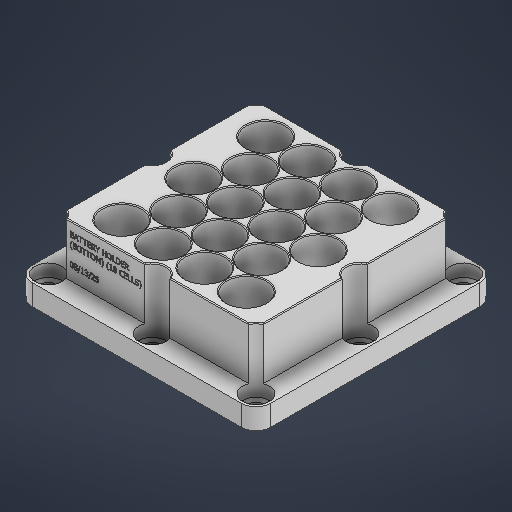
# Autodesk Inventor part: Battery Holder
Saved by Autodesk Inventor 2025 (Build 290162000, 162)
## iProperties
Created: 2025-08-08
Part Number: Battery Holder
Material: Generic
Document SubType Name: Modeling
Designer: mayhe
Density: 1 g/cm^3
Appearance: Default
Author: mayhe
Autodesk Inventor part; units mm, degrees
ref_plane "YZ Plane" through (0, 0, 0) normal (1, 0, 0) x (0, 1, 0)
ref_plane "XZ Plane" through (0, 0, 0) normal (0, 1, 0) x (-1, 0, 0)
ref_plane "XY Plane" through (0, 0, 0) normal (0, 0, 1) x (1, 0, 0)
sketch "Sketch1" plane through (0, 0, 0) normal (0, 1, 0) x (-1, 0, 0)
  line L0 (57.5, 57.5) -> (-57.5, 57.5)
  line L1 (-57.5, 57.5) -> (-57.5, -57.5)
  line L2 (-57.5, -57.5) -> (57.5, -57.5)
  line L3 (57.5, -57.5) -> (57.5, 57.5)
  line L4 (57.5, 57.5) -> (-57.5, -57.5) construction
  line L5 (-57.5, 57.5) -> (57.5, -57.5) construction
  point P0 (0, 0)
  dimension "d0" = 115
  dimension "d1" = 115
  constraints: 12 end point, 2 midpoint, 2 parallel, 1 horizontal, 1 perpendicular
  measures "d0" distance of L2.end L1.end
  measures "d1" distance of L1.end L0.end
extrude "Extrusion1" add sketch "Sketch1" along normal blind 10
sketch "Sketch4" plane through (0, 10, 0) normal (0, 1, 0) x (1, 0, 0)
  line L0 (-47.5, -47.5) -> (47.5, -47.5)
  line L1 (47.5, -47.5) -> (47.5, 47.5)
  line L2 (47.5, 47.5) -> (-47.5, 47.5)
  line L3 (-47.5, 47.5) -> (-47.5, -47.5)
  line L4 (-57.5, 57.5) -> (-57.5, -57.5) projected
  line L5 (-57.5, 0) -> (-47.5, 0)
  line L6 (-30, 34.641) -> (30, 34.641)
  line L7 (30, 34.641) -> (30, -34.641)
  line L8 (30, -34.641) -> (-30, -34.641)
  line L9 (-30, -34.641) -> (-30, 34.641)
  line L10 (-30, 34.641) -> (30, -34.641) construction
  line L11 (30, 34.641) -> (-30, -34.641) construction
  circle A0 centre (-30, 34.641) radius 9.5
  circle A1 centre (-10, 34.641) radius 9.5
  circle A2 centre (10, 34.641) radius 9.5
  circle A3 centre (30, 34.641) radius 9.5
  circle A4 centre (-30, 0) radius 9.5
  circle A5 centre (-10, 0) radius 9.5
  circle A6 centre (10, 0) radius 9.5
  circle A7 centre (30, 0) radius 9.5
  circle A8 centre (-30, -34.641) radius 9.5
  circle A9 centre (-10, -34.641) radius 9.5
  circle A10 centre (10, -34.641) radius 9.5
  circle A11 centre (30, -34.641) radius 9.5
  circle A12 centre (-20, 17.3205) radius 9.5
  circle A13 centre (0, 17.3205) radius 9.5
  circle A14 centre (20, 17.3205) radius 9.5
  circle A15 centre (-20, -17.3205) radius 9.5
  circle A16 centre (0, -17.3205) radius 9.5
  circle A17 centre (20, -17.3205) radius 9.5
  point P0 (47.3285, -94.6135)
  point P1 (-53.5957, 219.1108)
  point P2 (0, 0)
  dimension "d1" = 115
  dimension "d138" = 3
  dimension "d48" = 95
  dimension "d49" = 95
  dimension "d132" = 60
  dimension "d133" = 69.282
  dimension "d134" = 19
  dimension "d137" = 20
  dimension "d140" = 34.641
  dimension "d143" = 19
  dimension "d146" = 10
  dimension "d147" = 17.3205
  dimension "d150" = 20
  dimension "d153" = 34.641
  constraints: 22 end point, 18 centre point, 4 horizontal, 4 midpoint, 4 parallel, 2 perpendicular, 2 vertical, 1 coincident, 32 other
  measures "d48" distance of L2.end L1.end
  measures "d49" distance of L1.end L0.end
  measures "d132" distance of L7.end L8.end
  measures "d133" distance of L6.end L7.end
  measures "d134" diameter of A0
  measures "d137" distance of A0.centre A1.centre
  measures "d140" distance of A0.centre A4.centre
  measures "d143" diameter of A12
  measures "d146" horizontal distance of A1.centre A12.centre
  measures "d147" vertical distance of A12.centre A1.centre
  measures "d150" distance of A12.centre A13.centre
  measures "d153" distance of A12.centre A15.centre
extrude "Extrusion2" add sketch "Sketch4" along normal blind 25 contours L3 L2 L1 L0 | L6 A1 A2 A3 L7 A7 A11 L8 A10 A9 A8 L9 A4 A0
sketch "Sketch5" plane through (0, 35, 0) normal (0, 1, 0) x (1, 0, 0)
  line L0 (50, 50) -> (-50, 50)
  line L1 (-50, 50) -> (-50, -50)
  line L2 (-50, -50) -> (50, -50)
  line L3 (50, -50) -> (50, 50)
  line L4 (50, 50) -> (-50, -50) construction
  line L5 (-50, 50) -> (50, -50) construction
  circle A0 centre (-50, -50) radius 3.5
  circle A1 centre (0, -50) radius 3.5
  circle A2 centre (-50, 0) radius 3.5
  circle A3 centre (0, 0) radius 3.5
  circle A4 centre (50, -50) radius 3.5
  circle A5 centre (50, 0) radius 3.5
  circle A6 centre (-50, 50) radius 3.5
  circle A7 centre (0, 50) radius 3.5
  circle A8 centre (50, 50) radius 3.5
  point P0 (0, 0)
  dimension "d156" = 100
  dimension "d157" = 100
  dimension "d158" = 7
  dimension "d161" = 50
  dimension "d164" = 50
  constraints: 12 end point, 9 centre point, 2 horizontal, 2 midpoint, 2 parallel, 1 coincident, 1 perpendicular, 1 vertical, 16 other
  measures "d156" distance of L2.end L1.end
  measures "d157" distance of L1.end L0.end
  measures "d158" diameter of A0
  measures "d161" distance of A0.centre A1.centre
  measures "d164" distance of A0.centre A2.centre
hole "Hole3" at (-50, 35, 50) at (50, 35, 50) at (-50, 35, -50) at (50, 35, -50) at (-50, 35, 0) at (0, 35, 50) at (50, 35, 0) at (0, 35, -50) direction (0, -1, 0) diameter 7.125 end through all counterbore diameter 13 counterbore depth 31
fillet "Fillet1" radius 7.125 4 edges at (57.5, 5, 57.5) (57.5, 5, -57.5) (-57.5, 5, 57.5) (-57.5, 5, -57.5)
chamfer "Chamfer1" distance 0.4 angle 45 35 edges at (-39.5, 35, -34.641) (-19.5, 35, -34.641) (-29.5, 35, -17.3205) (0.5, 35, -34.641) (20.5, 35, -34.641) (10.5, 35, -17.3205) (-9.5, 35, -17.3205) (-39.5, 35, 0) (-19.5, 35, 0) (0.5, 35, 0) (20.5, 35, 0) (10.5, 35, 17.3205) (-9.5, 35, 17.3205) (-29.5, 35, 17.3205) (-39.5, 35, 34.641) (-19.5, 35, 34.641) (0.5, 35, 34.641) (20.5, 35, 34.641) (-25, 35, 47.5) (25, 35, 47.5) (0, 35, 43.5) (45.4038, 35, 45.4038) (47.5, 35, 25) (47.5, 35, -25) (43.5, 35, 0) (45.4038, 35, -45.4038) (25, 35, -47.5) (-25, 35, -47.5) (3.6056, 35, -44.5917) (-3.6056, 35, -44.5917) (-45.4038, 35, -45.4038) (-47.5, 35, -25) (-47.5, 35, 25) (-43.5, 35, 0) (-45.4038, 35, 45.4038)
sketch "Sketch6" plane through (-44, 10, 47.5) normal (0, 0, 1) x (1, 0, 0)
  line L0 (1.8145, 20.8005) -> (43.0895, 20.8005) construction
  line L1 (43.0895, 20.8005) -> (43.0895, -1.7911) construction
  line L2 (43.0895, -1.7911) -> (1.8145, -1.7911) construction
  line L3 (1.8145, -1.7911) -> (1.8145, 20.8005) construction
  spline S0 degree 2 poles (3.7946, 18.987) (3.7946, 18.7977) (3.6505, 18.5075) (3.5311, 18.4128) knots 0 0 0 1 2 2 2
  spline S1 degree 2 poles (3.5311, 18.4128) (3.387, 18.3016) (3.0598, 18.2069) (2.8004, 18.2069) knots 0 0 0 1 2 2 2
  line L4 (2.8004, 18.2069) -> (2.0717, 18.2069)
  line L5 (2.0717, 18.2069) -> (2.0717, 20.7469)
  line L6 (2.0717, 20.7469) -> (2.7448, 20.7469)
  spline S2 degree 2 poles (2.7448, 20.7469) (3.0165, 20.7469) (3.2882, 20.7119) (3.4117, 20.644) knots 0 0 0 1 2 2 2
  spline S3 degree 2 poles (3.4117, 20.644) (3.5496, 20.572) (3.6752, 20.3353) (3.6752, 20.1747) knots 0 0 0 1 2 2 2
  spline S4 degree 2 poles (3.6752, 20.1747) (3.6752, 19.9956) (3.4858, 19.7116) (3.3191, 19.6313) knots 0 0 0 1 2 2 2
  line L7 (3.3191, 19.6313) -> (3.3191, 19.619)
  spline S5 degree 2 poles (3.3191, 19.619) (3.5455, 19.5572) (3.7946, 19.2299) (3.7946, 18.987) knots 0 0 0 1 2 2 2
  spline S6 degree 2 poles (3.4426, 18.9726) (3.4426, 19.1167) (3.3603, 19.302) (3.2368, 19.3678) knots 0 0 0 1 2 2 2
  spline S7 degree 2 poles (3.2368, 19.3678) (3.1565, 19.409) (2.9671, 19.4337) (2.7922, 19.4337) knots 0 0 0 1 2 2 2
  line L8 (2.7922, 19.4337) -> (2.4093, 19.4337)
  line L9 (2.4093, 19.4337) -> (2.4093, 18.4951)
  line L10 (2.4093, 18.4951) -> (2.6831, 18.4951)
  spline S8 degree 2 poles (2.6831, 18.4951) (2.9054, 18.4951) (3.1606, 18.5363) (3.2594, 18.6021) knots 0 0 0 1 2 2 2
  spline S9 degree 2 poles (3.2594, 18.6021) (3.3541, 18.6701) (3.4426, 18.8388) (3.4426, 18.9726) knots 0 0 0 1 2 2 2
  spline S10 degree 2 poles (3.3232, 20.1274) (3.3232, 20.2179) (3.2615, 20.3538) (3.1935, 20.3929) knots 0 0 0 1 2 2 2
  spline S11 degree 2 poles (3.1935, 20.3929) (3.1112, 20.4382) (2.9116, 20.4588) (2.7325, 20.4588) knots 0 0 0 1 2 2 2
  line L11 (2.7325, 20.4588) -> (2.4093, 20.4588)
  line L12 (2.4093, 20.4588) -> (2.4093, 19.7157)
  line L13 (2.4093, 19.7157) -> (2.7922, 19.7157)
  spline S12 degree 2 poles (2.7922, 19.7157) (2.9507, 19.7157) (3.1009, 19.7486) (3.1812, 19.8001) knots 0 0 0 1 2 2 2
  spline S13 degree 2 poles (3.1812, 19.8001) (3.2594, 19.8495) (3.3232, 20.008) (3.3232, 20.1274) knots 0 0 0 1 2 2 2
  line L14 (3.8563, 18.2069) -> (4.7126, 20.7469)
  line L15 (4.7126, 20.7469) -> (5.1284, 20.7469)
  line L16 (5.1284, 20.7469) -> (5.9847, 18.2069)
  line L17 (5.9847, 18.2069) -> (5.6286, 18.2069)
  line L18 (5.6286, 18.2069) -> (5.398, 18.9171)
  line L19 (5.398, 18.9171) -> (4.4286, 18.9171)
  line L20 (4.4286, 18.9171) -> (4.198, 18.2069)
  line L21 (4.198, 18.2069) -> (3.8563, 18.2069)
  line L22 (5.3054, 19.2052) -> (4.9123, 20.4011)
  line L23 (4.9123, 20.4011) -> (4.5212, 19.2052)
  line L24 (4.5212, 19.2052) -> (5.3054, 19.2052)
  line L25 (6.8183, 18.2069) -> (6.8183, 20.4464)
  line L26 (6.8183, 20.4464) -> (5.9661, 20.4464)
  line L27 (5.9661, 20.4464) -> (5.9661, 20.7469)
  line L28 (5.9661, 20.7469) -> (8.008, 20.7469)
  line L29 (8.008, 20.7469) -> (8.008, 20.4464)
  line L30 (8.008, 20.4464) -> (7.1559, 20.4464)
  line L31 (7.1559, 20.4464) -> (7.1559, 18.2069)
  line L32 (7.1559, 18.2069) -> (6.8183, 18.2069)
  line L33 (8.8581, 18.2069) -> (8.8581, 20.4464)
  line L34 (8.8581, 20.4464) -> (8.006, 20.4464)
  line L35 (8.006, 20.4464) -> (8.006, 20.7469)
  line L36 (8.006, 20.7469) -> (10.0478, 20.7469)
  line L37 (10.0478, 20.7469) -> (10.0478, 20.4464)
  line L38 (10.0478, 20.4464) -> (9.1957, 20.4464)
  line L39 (9.1957, 20.4464) -> (9.1957, 18.2069)
  line L40 (9.1957, 18.2069) -> (8.8581, 18.2069)
  line L41 (10.3051, 18.2069) -> (10.3051, 20.7469)
  line L42 (10.3051, 20.7469) -> (11.8942, 20.7469)
  line L43 (11.8942, 20.7469) -> (11.8942, 20.4464)
  line L44 (11.8942, 20.4464) -> (10.6427, 20.4464)
  line L45 (10.6427, 20.4464) -> (10.6427, 19.7507)
  line L46 (10.6427, 19.7507) -> (11.8098, 19.7507)
  line L47 (11.8098, 19.7507) -> (11.8098, 19.4502)
  line L48 (11.8098, 19.4502) -> (10.6427, 19.4502)
  line L49 (10.6427, 19.4502) -> (10.6427, 18.5075)
  line L50 (10.6427, 18.5075) -> (11.8942, 18.5075)
  line L51 (11.8942, 18.5075) -> (11.8942, 18.2069)
  line L52 (11.8942, 18.2069) -> (10.3051, 18.2069)
  line L53 (14.2304, 18.2069) -> (13.792, 18.2069)
  line L54 (13.792, 18.2069) -> (12.9892, 19.2176)
  line L55 (12.9892, 19.2176) -> (12.6023, 19.2176)
  line L56 (12.6023, 19.2176) -> (12.6023, 18.2069)
  line L57 (12.6023, 18.2069) -> (12.2647, 18.2069)
  line L58 (12.2647, 18.2069) -> (12.2647, 20.7469)
  line L59 (12.2647, 20.7469) -> (12.9192, 20.7469)
  spline S14 degree 2 poles (12.9192, 20.7469) (13.1374, 20.7469) (13.4318, 20.6996) (13.5656, 20.6131) knots 0 0 0 1 2 2 2
  spline S15 degree 2 poles (13.5656, 20.6131) (13.6993, 20.5267) (13.8537, 20.257) (13.8537, 20.0574) knots 0 0 0 1 2 2 2
  spline S16 degree 2 poles (13.8537, 20.0574) (13.8537, 19.7795) (13.5697, 19.4028) (13.3268, 19.3123) knots 0 0 0 1 2 2 2
  line L60 (13.3268, 19.3123) -> (14.2304, 18.2069)
  spline S17 degree 2 poles (13.5017, 20.0306) (13.5017, 20.1418) (13.4235, 20.3126) (13.3412, 20.3682) knots 0 0 0 1 2 2 2
  spline S18 degree 2 poles (13.3412, 20.3682) (13.2692, 20.4155) (13.0777, 20.4547) (12.9378, 20.4547) knots 0 0 0 1 2 2 2
  line L61 (12.9378, 20.4547) -> (12.6023, 20.4547)
  line L62 (12.6023, 20.4547) -> (12.6023, 19.4996)
  line L63 (12.6023, 19.4996) -> (12.8987, 19.4996)
  spline S19 degree 2 poles (12.8987, 19.4996) (13.0448, 19.4996) (13.2774, 19.551) (13.3577, 19.6313) knots 0 0 0 1 2 2 2
  spline S20 degree 2 poles (13.3577, 19.6313) (13.4318, 19.7013) (13.5017, 19.8989) (13.5017, 20.0306) knots 0 0 0 1 2 2 2
  line L64 (16.2105, 20.7469) -> (15.3522, 19.3308)
  line L65 (15.3522, 19.3308) -> (15.3522, 18.2069)
  line L66 (15.3522, 18.2069) -> (15.0146, 18.2069)
  line L67 (15.0146, 18.2069) -> (15.0146, 19.2958)
  line L68 (15.0146, 19.2958) -> (14.1563, 20.7469)
  line L69 (14.1563, 20.7469) -> (14.5309, 20.7469)
  line L70 (14.5309, 20.7469) -> (15.1875, 19.6293)
  line L71 (15.1875, 19.6293) -> (15.8524, 20.7469)
  line L72 (15.8524, 20.7469) -> (16.2105, 20.7469)
  line L73 (19.3804, 18.2069) -> (19.0428, 18.2069)
  line L74 (19.0428, 18.2069) -> (19.0428, 19.4502)
  line L75 (19.0428, 19.4502) -> (17.8737, 19.4502)
  line L76 (17.8737, 19.4502) -> (17.8737, 18.2069)
  line L77 (17.8737, 18.2069) -> (17.5361, 18.2069)
  line L78 (17.5361, 18.2069) -> (17.5361, 20.7469)
  line L79 (17.5361, 20.7469) -> (17.8737, 20.7469)
  line L80 (17.8737, 20.7469) -> (17.8737, 19.7507)
  line L81 (17.8737, 19.7507) -> (19.0428, 19.7507)
  line L82 (19.0428, 19.7507) -> (19.0428, 20.7469)
  line L83 (19.0428, 20.7469) -> (19.3804, 20.7469)
  line L84 (19.3804, 20.7469) -> (19.3804, 18.2069)
  spline S21 degree 2 poles (21.6919, 20.4567) (21.836, 20.2879) (21.9965, 19.7939) (21.9965, 19.4769) knots 0 0 0 1 2 2 2
  spline S22 degree 2 poles (21.9965, 19.4769) (21.9965, 19.1682) (21.8401, 18.668) (21.6919, 18.4992) knots 0 0 0 1 2 2 2
  spline S23 degree 2 poles (21.6919, 18.4992) (21.5355, 18.3222) (21.1217, 18.1534) (20.8727, 18.1534) knots 0 0 0 1 2 2 2
  spline S24 degree 2 poles (20.8727, 18.1534) (20.6154, 18.1534) (20.2037, 18.3284) (20.0535, 18.4992) knots 0 0 0 1 2 2 2
  spline S25 degree 2 poles (20.0535, 18.4992) (19.9073, 18.668) (19.7509, 19.1641) (19.7509, 19.4769) knots 0 0 0 1 2 2 2
  spline S26 degree 2 poles (19.7509, 19.4769) (19.7509, 19.796) (19.9094, 20.2817) (20.0555, 20.4567) knots 0 0 0 1 2 2 2
  spline S27 degree 2 poles (20.0555, 20.4567) (20.2037, 20.6255) (20.6175, 20.8005) (20.8727, 20.8005) knots 0 0 0 1 2 2 2
  spline S28 degree 2 poles (20.8727, 20.8005) (21.132, 20.8005) (21.5478, 20.6193) (21.6919, 20.4567) knots 0 0 0 1 2 2 2
  spline S29 degree 2 poles (21.6446, 19.4769) (21.6446, 19.7281) (21.5355, 20.1171) (21.4367, 20.2447) knots 0 0 0 1 2 2 2
  spline S30 degree 2 poles (21.4367, 20.2447) (21.3358, 20.3764) (21.0518, 20.5082) (20.8747, 20.5082) knots 0 0 0 1 2 2 2
  spline S31 degree 2 poles (20.8747, 20.5082) (20.6916, 20.5082) (20.4157, 20.3806) (20.3108, 20.2447) knots 0 0 0 1 2 2 2
  spline S32 degree 2 poles (20.3108, 20.2447) (20.2099, 20.115) (20.1029, 19.7239) (20.1029, 19.4769) knots 0 0 0 1 2 2 2
  spline S33 degree 2 poles (20.1029, 19.4769) (20.1029, 18.9768) (20.5228, 18.4457) (20.8747, 18.4457) knots 0 0 0 1 2 2 2
  spline S34 degree 2 poles (20.8747, 18.4457) (21.2267, 18.4457) (21.6446, 18.9768) (21.6446, 19.4769) knots 0 0 0 1 2 2 2
  line L85 (23.8388, 18.2069) -> (22.367, 18.2069)
  line L86 (22.367, 18.2069) -> (22.367, 20.7469)
  line L87 (22.367, 20.7469) -> (22.7046, 20.7469)
  line L88 (22.7046, 20.7469) -> (22.7046, 18.5075)
  line L89 (22.7046, 18.5075) -> (23.8388, 18.5075)
  line L90 (23.8388, 18.5075) -> (23.8388, 18.2069)
  spline S35 degree 2 poles (26.1071, 19.4749) (26.1071, 19.127) (25.8251, 18.5671) (25.5884, 18.4107) knots 0 0 0 1 2 2 2
  spline S36 degree 2 poles (25.5884, 18.4107) (25.3949, 18.2893) (24.9976, 18.2069) (24.6889, 18.2069) knots 0 0 0 1 2 2 2
  line L91 (24.6889, 18.2069) -> (24.1043, 18.2069)
  line L92 (24.1043, 18.2069) -> (24.1043, 20.7469)
  line L93 (24.1043, 20.7469) -> (24.6827, 20.7469)
  spline S37 degree 2 poles (24.6827, 20.7469) (25.0408, 20.7469) (25.4484, 20.6399) (25.5925, 20.5452) knots 0 0 0 1 2 2 2
  spline S38 degree 2 poles (25.5925, 20.5452) (25.8374, 20.3826) (26.1071, 19.8454) (26.1071, 19.4749) knots 0 0 0 1 2 2 2
  spline S39 degree 2 poles (25.7551, 19.479) (25.7551, 19.7713) (25.5616, 20.185) (25.3702, 20.3023) knots 0 0 0 1 2 2 2
  spline S40 degree 2 poles (25.3702, 20.3023) (25.2343, 20.3826) (24.9276, 20.4547) (24.6992, 20.4547) knots 0 0 0 1 2 2 2
  line L94 (24.6992, 20.4547) -> (24.4419, 20.4547)
  line L95 (24.4419, 20.4547) -> (24.4419, 18.4992)
  line L96 (24.4419, 18.4992) -> (24.6992, 18.4992)
  spline S41 degree 2 poles (24.6992, 18.4992) (24.9235, 18.4992) (25.2631, 18.5713) (25.4011, 18.668) knots 0 0 0 1 2 2 2
  spline S42 degree 2 poles (25.4011, 18.668) (25.5781, 18.7874) (25.7551, 19.1826) (25.7551, 19.479) knots 0 0 0 1 2 2 2
  line L97 (26.4735, 18.2069) -> (26.4735, 20.7469)
  line L98 (26.4735, 20.7469) -> (28.0625, 20.7469)
  line L99 (28.0625, 20.7469) -> (28.0625, 20.4464)
  line L100 (28.0625, 20.4464) -> (26.811, 20.4464)
  line L101 (26.811, 20.4464) -> (26.811, 19.7507)
  line L102 (26.811, 19.7507) -> (27.9781, 19.7507)
  line L103 (27.9781, 19.7507) -> (27.9781, 19.4502)
  line L104 (27.9781, 19.4502) -> (26.811, 19.4502)
  line L105 (26.811, 19.4502) -> (26.811, 18.5075)
  line L106 (26.811, 18.5075) -> (28.0625, 18.5075)
  line L107 (28.0625, 18.5075) -> (28.0625, 18.2069)
  line L108 (28.0625, 18.2069) -> (26.4735, 18.2069)
  line L109 (30.3987, 18.2069) -> (29.9603, 18.2069)
  line L110 (29.9603, 18.2069) -> (29.1575, 19.2176)
  line L111 (29.1575, 19.2176) -> (28.7706, 19.2176)
  line L112 (28.7706, 19.2176) -> (28.7706, 18.2069)
  line L113 (28.7706, 18.2069) -> (28.433, 18.2069)
  line L114 (28.433, 18.2069) -> (28.433, 20.7469)
  line L115 (28.433, 20.7469) -> (29.0876, 20.7469)
  spline S43 degree 2 poles (29.0876, 20.7469) (29.3057, 20.7469) (29.6001, 20.6996) (29.7339, 20.6131) knots 0 0 0 1 2 2 2
  spline S44 degree 2 poles (29.7339, 20.6131) (29.8677, 20.5267) (30.022, 20.257) (30.022, 20.0574) knots 0 0 0 1 2 2 2
  spline S45 degree 2 poles (30.022, 20.0574) (30.022, 19.7795) (29.738, 19.4028) (29.4951, 19.3123) knots 0 0 0 1 2 2 2
  line L116 (29.4951, 19.3123) -> (30.3987, 18.2069)
  spline S46 degree 2 poles (29.6701, 20.0306) (29.6701, 20.1418) (29.5918, 20.3126) (29.5095, 20.3682) knots 0 0 0 1 2 2 2
  spline S47 degree 2 poles (29.5095, 20.3682) (29.4375, 20.4155) (29.246, 20.4547) (29.1061, 20.4547) knots 0 0 0 1 2 2 2
  line L117 (29.1061, 20.4547) -> (28.7706, 20.4547)
  line L118 (28.7706, 20.4547) -> (28.7706, 19.4996)
  line L119 (28.7706, 19.4996) -> (29.067, 19.4996)
  spline S48 degree 2 poles (29.067, 19.4996) (29.2131, 19.4996) (29.4457, 19.551) (29.526, 19.6313) knots 0 0 0 1 2 2 2
  spline S49 degree 2 poles (29.526, 19.6313) (29.6001, 19.7013) (29.6701, 19.8989) (29.6701, 20.0306) knots 0 0 0 1 2 2 2
  line L120 (3.0248, 13.323) -> (2.6337, 13.323)
  spline S50 degree 2 poles (2.6337, 13.323) (2.3373, 13.675) (1.9976, 14.4633) (1.9976, 15.0005) knots 0 0 0 1 2 2 2
  spline S51 degree 2 poles (1.9976, 15.0005) (1.9976, 15.5254) (2.3332, 16.3261) (2.6337, 16.6781) knots 0 0 0 1 2 2 2
  line L121 (2.6337, 16.6781) -> (3.0248, 16.6781)
  line L122 (3.0248, 16.6781) -> (3.0248, 16.6616)
  spline S52 degree 2 poles (3.0248, 16.6616) (2.8869, 16.5361) (2.6357, 16.2109) (2.5287, 15.9947) knots 0 0 0 1 2 2 2
  spline S53 degree 2 poles (2.5287, 15.9947) (2.4258, 15.7848) (2.2982, 15.2805) (2.2982, 15.0005) knots 0 0 0 1 2 2 2
  spline S54 degree 2 poles (2.2982, 15.0005) (2.2982, 14.7083) (2.4217, 14.2246) (2.5287, 14.0064) knots 0 0 0 1 2 2 2
  spline S55 degree 2 poles (2.5287, 14.0064) (2.6316, 13.7964) (2.893, 13.4568) (3.0248, 13.3395) knots 0 0 0 1 2 2 2
  line L123 (3.0248, 13.3395) -> (3.0248, 13.323)
  spline S56 degree 2 poles (5.1325, 14.805) (5.1325, 14.6156) (4.9884, 14.3254) (4.869, 14.2307) knots 0 0 0 1 2 2 2
  spline S57 degree 2 poles (4.869, 14.2307) (4.725, 14.1196) (4.3977, 14.0249) (4.1383, 14.0249) knots 0 0 0 1 2 2 2
  line L124 (4.1383, 14.0249) -> (3.4097, 14.0249)
  line L125 (3.4097, 14.0249) -> (3.4097, 16.5649)
  line L126 (3.4097, 16.5649) -> (4.0828, 16.5649)
  spline S58 degree 2 poles (4.0828, 16.5649) (4.3545, 16.5649) (4.6262, 16.5299) (4.7497, 16.462) knots 0 0 0 1 2 2 2
  spline S59 degree 2 poles (4.7497, 16.462) (4.8876, 16.3899) (5.0131, 16.1532) (5.0131, 15.9927) knots 0 0 0 1 2 2 2
  spline S60 degree 2 poles (5.0131, 15.9927) (5.0131, 15.8136) (4.8238, 15.5295) (4.657, 15.4493) knots 0 0 0 1 2 2 2
  line L127 (4.657, 15.4493) -> (4.657, 15.4369)
  spline S61 degree 2 poles (4.657, 15.4369) (4.8835, 15.3752) (5.1325, 15.0479) (5.1325, 14.805) knots 0 0 0 1 2 2 2
  spline S62 degree 2 poles (4.7805, 14.7906) (4.7805, 14.9347) (4.6982, 15.1199) (4.5747, 15.1858) knots 0 0 0 1 2 2 2
  spline S63 degree 2 poles (4.5747, 15.1858) (4.4944, 15.227) (4.3051, 15.2517) (4.1301, 15.2517) knots 0 0 0 1 2 2 2
  line L128 (4.1301, 15.2517) -> (3.7472, 15.2517)
  line L129 (3.7472, 15.2517) -> (3.7472, 14.3131)
  line L130 (3.7472, 14.3131) -> (4.021, 14.3131)
  spline S64 degree 2 poles (4.021, 14.3131) (4.2433, 14.3131) (4.4985, 14.3542) (4.5973, 14.4201) knots 0 0 0 1 2 2 2
  spline S65 degree 2 poles (4.5973, 14.4201) (4.692, 14.488) (4.7805, 14.6568) (4.7805, 14.7906) knots 0 0 0 1 2 2 2
  spline S66 degree 2 poles (4.6611, 15.9453) (4.6611, 16.0359) (4.5994, 16.1717) (4.5315, 16.2109) knots 0 0 0 1 2 2 2
  spline S67 degree 2 poles (4.5315, 16.2109) (4.4491, 16.2561) (4.2495, 16.2767) (4.0704, 16.2767) knots 0 0 0 1 2 2 2
  line L131 (4.0704, 16.2767) -> (3.7472, 16.2767)
  line L132 (3.7472, 16.2767) -> (3.7472, 15.5337)
  line L133 (3.7472, 15.5337) -> (4.1301, 15.5337)
  spline S68 degree 2 poles (4.1301, 15.5337) (4.2886, 15.5337) (4.4388, 15.5666) (4.5191, 15.6181) knots 0 0 0 1 2 2 2
  spline S69 degree 2 poles (4.5191, 15.6181) (4.5973, 15.6675) (4.6611, 15.8259) (4.6611, 15.9453) knots 0 0 0 1 2 2 2
  spline S70 degree 2 poles (7.265, 16.2747) (7.409, 16.1059) (7.5696, 15.6119) (7.5696, 15.2949) knots 0 0 0 1 2 2 2
  spline S71 degree 2 poles (7.5696, 15.2949) (7.5696, 14.9861) (7.4132, 14.486) (7.265, 14.3172) knots 0 0 0 1 2 2 2
  spline S72 degree 2 poles (7.265, 14.3172) (7.1085, 14.1402) (6.6948, 13.9714) (6.4457, 13.9714) knots 0 0 0 1 2 2 2
  spline S73 degree 2 poles (6.4457, 13.9714) (6.1884, 13.9714) (5.7768, 14.1463) (5.6265, 14.3172) knots 0 0 0 1 2 2 2
  spline S74 degree 2 poles (5.6265, 14.3172) (5.4804, 14.486) (5.3239, 14.982) (5.3239, 15.2949) knots 0 0 0 1 2 2 2
  spline S75 degree 2 poles (5.3239, 15.2949) (5.3239, 15.6139) (5.4824, 16.0997) (5.6286, 16.2747) knots 0 0 0 1 2 2 2
  spline S76 degree 2 poles (5.6286, 16.2747) (5.7768, 16.4435) (6.1905, 16.6184) (6.4457, 16.6184) knots 0 0 0 1 2 2 2
  spline S77 degree 2 poles (6.4457, 16.6184) (6.7051, 16.6184) (7.1209, 16.4373) (7.265, 16.2747) knots 0 0 0 1 2 2 2
  spline S78 degree 2 poles (7.2176, 15.2949) (7.2176, 15.546) (7.1085, 15.935) (7.0097, 16.0627) knots 0 0 0 1 2 2 2
  spline S79 degree 2 poles (7.0097, 16.0627) (6.9089, 16.1944) (6.6248, 16.3261) (6.4478, 16.3261) knots 0 0 0 1 2 2 2
  spline S80 degree 2 poles (6.4478, 16.3261) (6.2646, 16.3261) (5.9888, 16.1985) (5.8838, 16.0627) knots 0 0 0 1 2 2 2
  spline S81 degree 2 poles (5.8838, 16.0627) (5.7829, 15.933) (5.6759, 15.5419) (5.6759, 15.2949) knots 0 0 0 1 2 2 2
  spline S82 degree 2 poles (5.6759, 15.2949) (5.6759, 14.7947) (6.0958, 14.2637) (6.4478, 14.2637) knots 0 0 0 1 2 2 2
  spline S83 degree 2 poles (6.4478, 14.2637) (6.7998, 14.2637) (7.2176, 14.7947) (7.2176, 15.2949) knots 0 0 0 1 2 2 2
  line L134 (8.5329, 14.0249) -> (8.5329, 16.2644)
  line L135 (8.5329, 16.2644) -> (7.6807, 16.2644)
  line L136 (7.6807, 16.2644) -> (7.6807, 16.5649)
  line L137 (7.6807, 16.5649) -> (9.7226, 16.5649)
  line L138 (9.7226, 16.5649) -> (9.7226, 16.2644)
  line L139 (9.7226, 16.2644) -> (8.8705, 16.2644)
  line L140 (8.8705, 16.2644) -> (8.8705, 14.0249)
  line L141 (8.8705, 14.0249) -> (8.5329, 14.0249)
  line L142 (10.5727, 14.0249) -> (10.5727, 16.2644)
  line L143 (10.5727, 16.2644) -> (9.7206, 16.2644)
  line L144 (9.7206, 16.2644) -> (9.7206, 16.5649)
  line L145 (9.7206, 16.5649) -> (11.7624, 16.5649)
  line L146 (11.7624, 16.5649) -> (11.7624, 16.2644)
  line L147 (11.7624, 16.2644) -> (10.9103, 16.2644)
  line L148 (10.9103, 16.2644) -> (10.9103, 14.0249)
  line L149 (10.9103, 14.0249) -> (10.5727, 14.0249)
  spline S84 degree 2 poles (13.8167, 16.2747) (13.9608, 16.1059) (14.1213, 15.6119) (14.1213, 15.2949) knots 0 0 0 1 2 2 2
  spline S85 degree 2 poles (14.1213, 15.2949) (14.1213, 14.9861) (13.9649, 14.486) (13.8167, 14.3172) knots 0 0 0 1 2 2 2
  spline S86 degree 2 poles (13.8167, 14.3172) (13.6602, 14.1402) (13.2465, 13.9714) (12.9975, 13.9714) knots 0 0 0 1 2 2 2
  spline S87 degree 2 poles (12.9975, 13.9714) (12.7402, 13.9714) (12.3285, 14.1463) (12.1782, 14.3172) knots 0 0 0 1 2 2 2
  spline S88 degree 2 poles (12.1782, 14.3172) (12.0321, 14.486) (11.8757, 14.982) (11.8757, 15.2949) knots 0 0 0 1 2 2 2
  spline S89 degree 2 poles (11.8757, 15.2949) (11.8757, 15.6139) (12.0341, 16.0997) (12.1803, 16.2747) knots 0 0 0 1 2 2 2
  spline S90 degree 2 poles (12.1803, 16.2747) (12.3285, 16.4435) (12.7422, 16.6184) (12.9975, 16.6184) knots 0 0 0 1 2 2 2
  spline S91 degree 2 poles (12.9975, 16.6184) (13.2568, 16.6184) (13.6726, 16.4373) (13.8167, 16.2747) knots 0 0 0 1 2 2 2
  spline S92 degree 2 poles (13.7693, 15.2949) (13.7693, 15.546) (13.6602, 15.935) (13.5614, 16.0627) knots 0 0 0 1 2 2 2
  spline S93 degree 2 poles (13.5614, 16.0627) (13.4606, 16.1944) (13.1765, 16.3261) (12.9995, 16.3261) knots 0 0 0 1 2 2 2
  spline S94 degree 2 poles (12.9995, 16.3261) (12.8163, 16.3261) (12.5405, 16.1985) (12.4355, 16.0627) knots 0 0 0 1 2 2 2
  spline S95 degree 2 poles (12.4355, 16.0627) (12.3347, 15.933) (12.2276, 15.5419) (12.2276, 15.2949) knots 0 0 0 1 2 2 2
  spline S96 degree 2 poles (12.2276, 15.2949) (12.2276, 14.7947) (12.6475, 14.2637) (12.9995, 14.2637) knots 0 0 0 1 2 2 2
  spline S97 degree 2 poles (12.9995, 14.2637) (13.3515, 14.2637) (13.7693, 14.7947) (13.7693, 15.2949) knots 0 0 0 1 2 2 2
  line L150 (16.6695, 14.0249) -> (16.332, 14.0249)
  line L151 (16.332, 14.0249) -> (16.332, 16.2129)
  line L152 (16.332, 16.2129) -> (15.6692, 14.7247)
  line L153 (15.6692, 14.7247) -> (15.4634, 14.7247)
  line L154 (15.4634, 14.7247) -> (14.8067, 16.2129)
  line L155 (14.8067, 16.2129) -> (14.8067, 14.0249)
  line L156 (14.8067, 14.0249) -> (14.4918, 14.0249)
  line L157 (14.4918, 14.0249) -> (14.4918, 16.5649)
  line L158 (14.4918, 16.5649) -> (14.9529, 16.5649)
  line L159 (14.9529, 16.5649) -> (15.5869, 15.1508)
  line L160 (15.5869, 15.1508) -> (16.2002, 16.5649)
  line L161 (16.2002, 16.5649) -> (16.6695, 16.5649)
  line L162 (16.6695, 16.5649) -> (16.6695, 14.0249)
  spline S98 degree 2 poles (18.0816, 15.0005) (18.0816, 14.4736) (17.744, 13.675) (17.4455, 13.323) knots 0 0 0 1 2 2 2
  line L163 (17.4455, 13.323) -> (17.0545, 13.323)
  line L164 (17.0545, 13.323) -> (17.0545, 13.3395)
  spline S99 degree 2 poles (17.0545, 13.3395) (17.1862, 13.4568) (17.4517, 13.8005) (17.5505, 14.0064) knots 0 0 0 1 2 2 2
  spline S100 degree 2 poles (17.5505, 14.0064) (17.6576, 14.2266) (17.7811, 14.7165) (17.7811, 15.0005) knots 0 0 0 1 2 2 2
  spline S101 degree 2 poles (17.7811, 15.0005) (17.7811, 15.2825) (17.6555, 15.7827) (17.5505, 15.9947) knots 0 0 0 1 2 2 2
  spline S102 degree 2 poles (17.5505, 15.9947) (17.4476, 16.2067) (17.1841, 16.5443) (17.0545, 16.6616) knots 0 0 0 1 2 2 2
  line L165 (17.0545, 16.6616) -> (17.0545, 16.6781)
  line L166 (17.0545, 16.6781) -> (17.4455, 16.6781)
  spline S103 degree 2 poles (17.4455, 16.6781) (17.7419, 16.3261) (18.0816, 15.5316) (18.0816, 15.0005) knots 0 0 0 1 2 2 2
  line L167 (20.566, 13.323) -> (20.1749, 13.323)
  spline S104 degree 2 poles (20.1749, 13.323) (19.8785, 13.675) (19.5389, 14.4633) (19.5389, 15.0005) knots 0 0 0 1 2 2 2
  spline S105 degree 2 poles (19.5389, 15.0005) (19.5389, 15.5254) (19.8744, 16.3261) (20.1749, 16.6781) knots 0 0 0 1 2 2 2
  line L168 (20.1749, 16.6781) -> (20.566, 16.6781)
  line L169 (20.566, 16.6781) -> (20.566, 16.6616)
  spline S106 degree 2 poles (20.566, 16.6616) (20.4281, 16.5361) (20.177, 16.2109) (20.0699, 15.9947) knots 0 0 0 1 2 2 2
  spline S107 degree 2 poles (20.0699, 15.9947) (19.967, 15.7848) (19.8394, 15.2805) (19.8394, 15.0005) knots 0 0 0 1 2 2 2
  spline S108 degree 2 poles (19.8394, 15.0005) (19.8394, 14.7083) (19.9629, 14.2246) (20.0699, 14.0064) knots 0 0 0 1 2 2 2
  spline S109 degree 2 poles (20.0699, 14.0064) (20.1729, 13.7964) (20.4343, 13.4568) (20.566, 13.3395) knots 0 0 0 1 2 2 2
  line L170 (20.566, 13.3395) -> (20.566, 13.323)
  line L171 (22.3176, 14.0249) -> (21.0785, 14.0249)
  line L172 (21.0785, 14.0249) -> (21.0785, 14.2842)
  line L173 (21.0785, 14.2842) -> (21.5396, 14.2842)
  line L174 (21.5396, 14.2842) -> (21.5396, 15.9865)
  line L175 (21.5396, 15.9865) -> (21.0785, 15.9865)
  line L176 (21.0785, 15.9865) -> (21.0785, 16.2191)
  spline S110 degree 2 poles (21.0785, 16.2191) (21.3399, 16.2191) (21.5869, 16.3673) (21.6034, 16.5731) knots 0 0 0 1 2 2 2
  line L177 (21.6034, 16.5731) -> (21.8669, 16.5731)
  line L178 (21.8669, 16.5731) -> (21.8669, 14.2842)
  line L179 (21.8669, 14.2842) -> (22.3176, 14.2842)
  line L180 (22.3176, 14.2842) -> (22.3176, 14.0249)
  spline S111 degree 2 poles (23.5527, 13.9673) (23.3633, 13.9673) (23.0525, 14.0805) (22.9434, 14.1854) knots 0 0 0 1 2 2 2
  spline S112 degree 2 poles (22.9434, 14.1854) (22.8364, 14.2884) (22.7252, 14.5683) (22.7252, 14.7268) knots 0 0 0 1 2 2 2
  spline S113 degree 2 poles (22.7252, 14.7268) (22.7252, 14.9326) (22.9454, 15.2784) (23.1554, 15.3813) knots 0 0 0 1 2 2 2
  line L181 (23.1554, 15.3813) -> (23.1554, 15.3916)
  spline S114 degree 2 poles (23.1554, 15.3916) (22.9681, 15.5007) (22.787, 15.7601) (22.787, 15.9536) knots 0 0 0 1 2 2 2
  spline S115 degree 2 poles (22.787, 15.9536) (22.787, 16.2397) (23.2192, 16.6225) (23.5527, 16.6225) knots 0 0 0 1 2 2 2
  spline S116 degree 2 poles (23.5527, 16.6225) (23.8985, 16.6225) (24.3163, 16.2603) (24.3163, 15.9762) knots 0 0 0 1 2 2 2
  spline S117 degree 2 poles (24.3163, 15.9762) (24.3163, 15.8054) (24.1166, 15.4719) (23.9293, 15.3772) knots 0 0 0 1 2 2 2
  line L182 (23.9293, 15.3772) -> (23.9293, 15.3669)
  spline S118 degree 2 poles (23.9293, 15.3669) (24.1516, 15.264) (24.3801, 14.9676) (24.3801, 14.733) knots 0 0 0 1 2 2 2
  spline S119 degree 2 poles (24.3801, 14.733) (24.3801, 14.4077) (23.9067, 13.9673) (23.5527, 13.9673) knots 0 0 0 1 2 2 2
  spline S120 degree 2 poles (24.0302, 14.7) (24.0302, 14.8565) (23.9067, 15.0417) (23.7317, 15.1364) knots 0 0 0 1 2 2 2
  spline S121 degree 2 poles (23.7317, 15.1364) (23.6741, 15.1693) (23.4806, 15.2455) (23.3592, 15.2949) knots 0 0 0 1 2 2 2
  spline S122 degree 2 poles (23.3592, 15.2949) (23.2192, 15.2023) (23.0689, 14.9264) (23.0689, 14.7515) knots 0 0 0 1 2 2 2
  spline S123 degree 2 poles (23.0689, 14.7515) (23.0689, 14.521) (23.3468, 14.2204) (23.5568, 14.2204) knots 0 0 0 1 2 2 2
  spline S124 degree 2 poles (23.5568, 14.2204) (23.7708, 14.2204) (24.0302, 14.4777) (24.0302, 14.7) knots 0 0 0 1 2 2 2
  spline S125 degree 2 poles (23.9829, 15.9721) (23.9829, 16.1429) (23.7544, 16.3714) (23.5506, 16.3714) knots 0 0 0 1 2 2 2
  spline S126 degree 2 poles (23.5506, 16.3714) (23.3653, 16.3714) (23.1286, 16.1676) (23.1286, 15.9927) knots 0 0 0 1 2 2 2
  spline S127 degree 2 poles (23.1286, 15.9927) (23.1286, 15.8671) (23.2501, 15.6922) (23.3715, 15.6222) knots 0 0 0 1 2 2 2
  spline S128 degree 2 poles (23.3715, 15.6222) (23.423, 15.5934) (23.6412, 15.4925) (23.7297, 15.4637) knots 0 0 0 1 2 2 2
  spline S129 degree 2 poles (23.7297, 15.4637) (23.8779, 15.5769) (23.9829, 15.8177) (23.9829, 15.9721) knots 0 0 0 1 2 2 2
  spline S130 degree 2 poles (26.846, 13.9796) (26.599, 13.9796) (26.1812, 14.1463) (26.0288, 14.3131) knots 0 0 0 1 2 2 2
  spline S131 degree 2 poles (26.0288, 14.3131) (25.8765, 14.4777) (25.7098, 14.9717) (25.7098, 15.2928) knots 0 0 0 1 2 2 2
  spline S132 degree 2 poles (25.7098, 15.2928) (25.7098, 15.6119) (25.8724, 16.0853) (26.0268, 16.2603) knots 0 0 0 1 2 2 2
  spline S133 degree 2 poles (26.0268, 16.2603) (26.1791, 16.4311) (26.5949, 16.6102) (26.8522, 16.6102) knots 0 0 0 1 2 2 2
  spline S134 degree 2 poles (26.8522, 16.6102) (26.9798, 16.6102) (27.2042, 16.5731) (27.2988, 16.5443) knots 0 0 0 1 2 2 2
  spline S135 degree 2 poles (27.2988, 16.5443) (27.3812, 16.5176) (27.552, 16.4414) (27.6364, 16.3961) knots 0 0 0 1 2 2 2
  line L183 (27.6364, 16.3961) -> (27.6364, 15.9886)
  line L184 (27.6364, 15.9886) -> (27.6097, 15.9886)
  spline S136 degree 2 poles (27.6097, 15.9886) (27.5644, 16.0297) (27.4244, 16.145) (27.3235, 16.2006) knots 0 0 0 1 2 2 2
  spline S137 degree 2 poles (27.3235, 16.2006) (27.2268, 16.2541) (26.9983, 16.322) (26.8501, 16.322) knots 0 0 0 1 2 2 2
  spline S138 degree 2 poles (26.8501, 16.322) (26.6875, 16.322) (26.3973, 16.1882) (26.2882, 16.0606) knots 0 0 0 1 2 2 2
  spline S139 degree 2 poles (26.2882, 16.0606) (26.1812, 15.9309) (26.0618, 15.5378) (26.0618, 15.2928) knots 0 0 0 1 2 2 2
  spline S140 degree 2 poles (26.0618, 15.2928) (26.0618, 15.0314) (26.1873, 14.6547) (26.2964, 14.5251) knots 0 0 0 1 2 2 2
  spline S141 degree 2 poles (26.2964, 14.5251) (26.4035, 14.3995) (26.6896, 14.2719) (26.8501, 14.2719) knots 0 0 0 1 2 2 2
  spline S142 degree 2 poles (26.8501, 14.2719) (26.9963, 14.2719) (27.2453, 14.3439) (27.3421, 14.3975) knots 0 0 0 1 2 2 2
  spline S143 degree 2 poles (27.3421, 14.3975) (27.4347, 14.451) (27.5726, 14.5621) (27.6117, 14.6012) knots 0 0 0 1 2 2 2
  line L185 (27.6117, 14.6012) -> (27.6364, 14.6012)
  line L186 (27.6364, 14.6012) -> (27.6364, 14.1978)
  spline S144 degree 2 poles (27.6364, 14.1978) (27.552, 14.1587) (27.4038, 14.0866) (27.2988, 14.0537) knots 0 0 0 1 2 2 2
  spline S145 degree 2 poles (27.2988, 14.0537) (27.1877, 14.0167) (26.9983, 13.9796) (26.846, 13.9796) knots 0 0 0 1 2 2 2
  line L187 (27.9513, 14.0249) -> (27.9513, 16.5649)
  line L188 (27.9513, 16.5649) -> (29.5404, 16.5649)
  line L189 (29.5404, 16.5649) -> (29.5404, 16.2644)
  line L190 (29.5404, 16.2644) -> (28.2889, 16.2644)
  line L191 (28.2889, 16.2644) -> (28.2889, 15.5687)
  line L192 (28.2889, 15.5687) -> (29.456, 15.5687)
  line L193 (29.456, 15.5687) -> (29.456, 15.2681)
  line L194 (29.456, 15.2681) -> (28.2889, 15.2681)
  line L195 (28.2889, 15.2681) -> (28.2889, 14.3254)
  line L196 (28.2889, 14.3254) -> (29.5404, 14.3254)
  line L197 (29.5404, 14.3254) -> (29.5404, 14.0249)
  line L198 (29.5404, 14.0249) -> (27.9513, 14.0249)
  line L199 (31.3826, 14.0249) -> (29.9109, 14.0249)
  line L200 (29.9109, 14.0249) -> (29.9109, 16.5649)
  line L201 (29.9109, 16.5649) -> (30.2485, 16.5649)
  line L202 (30.2485, 16.5649) -> (30.2485, 14.3254)
  line L203 (30.2485, 14.3254) -> (31.3826, 14.3254)
  line L204 (31.3826, 14.3254) -> (31.3826, 14.0249)
  line L205 (33.1199, 14.0249) -> (31.6481, 14.0249)
  line L206 (31.6481, 14.0249) -> (31.6481, 16.5649)
  line L207 (31.6481, 16.5649) -> (31.9857, 16.5649)
  line L208 (31.9857, 16.5649) -> (31.9857, 14.3254)
  line L209 (31.9857, 14.3254) -> (33.1199, 14.3254)
  line L210 (33.1199, 14.3254) -> (33.1199, 14.0249)
  spline S146 degree 2 poles (34.0935, 13.9796) (33.8176, 13.9796) (33.4307, 14.0949) (33.2598, 14.1772) knots 0 0 0 1 2 2 2
  line L211 (33.2598, 14.1772) -> (33.2598, 14.6012)
  line L212 (33.2598, 14.6012) -> (33.2845, 14.6012)
  spline S147 degree 2 poles (33.2845, 14.6012) (33.4512, 14.4448) (33.8732, 14.2719) (34.0688, 14.2719) knots 0 0 0 1 2 2 2
  spline S148 degree 2 poles (34.0688, 14.2719) (34.3487, 14.2719) (34.6348, 14.5045) (34.6348, 14.6959) knots 0 0 0 1 2 2 2
  spline S149 degree 2 poles (34.6348, 14.6959) (34.6348, 14.8482) (34.4845, 15.0376) (34.3219, 15.0849) knots 0 0 0 1 2 2 2
  spline S150 degree 2 poles (34.3219, 15.0849) (34.2046, 15.1179) (34.0091, 15.1632) (33.8629, 15.2002) knots 0 0 0 1 2 2 2
  spline S151 degree 2 poles (33.8629, 15.2002) (33.7312, 15.2352) (33.5233, 15.3402) (33.443, 15.4246) knots 0 0 0 1 2 2 2
  spline S152 degree 2 poles (33.443, 15.4246) (33.3648, 15.509) (33.2783, 15.7354) (33.2783, 15.8836) knots 0 0 0 1 2 2 2
  spline S153 degree 2 poles (33.2783, 15.8836) (33.2783, 16.1923) (33.76, 16.6102) (34.1326, 16.6102) knots 0 0 0 1 2 2 2
  spline S154 degree 2 poles (34.1326, 16.6102) (34.3466, 16.6102) (34.7254, 16.5258) (34.888, 16.4455) knots 0 0 0 1 2 2 2
  line L213 (34.888, 16.4455) -> (34.888, 16.0421)
  line L214 (34.888, 16.0421) -> (34.8633, 16.0421)
  spline S155 degree 2 poles (34.8633, 16.0421) (34.7418, 16.1532) (34.3631, 16.3179) (34.1552, 16.3179) knots 0 0 0 1 2 2 2
  spline S156 degree 2 poles (34.1552, 16.3179) (33.9205, 16.3179) (33.6303, 16.0976) (33.6303, 15.9186) knots 0 0 0 1 2 2 2
  spline S157 degree 2 poles (33.6303, 15.9186) (33.6303, 15.758) (33.8012, 15.5666) (33.9617, 15.5234) knots 0 0 0 1 2 2 2
  spline S158 degree 2 poles (33.9617, 15.5234) (34.0688, 15.4946) (34.3796, 15.4205) (34.4825, 15.3896) knots 0 0 0 1 2 2 2
  spline S159 degree 2 poles (34.4825, 15.3896) (34.7439, 15.3093) (34.9868, 14.9861) (34.9868, 14.7494) knots 0 0 0 1 2 2 2
  spline S160 degree 2 poles (34.9868, 14.7494) (34.9868, 14.5992) (34.8653, 14.311) (34.7562, 14.2101) knots 0 0 0 1 2 2 2
  spline S161 degree 2 poles (34.7562, 14.2101) (34.6348, 14.099) (34.326, 13.9796) (34.0935, 13.9796) knots 0 0 0 1 2 2 2
  spline S162 degree 2 poles (36.228, 15.0005) (36.228, 14.4736) (35.8904, 13.675) (35.5919, 13.323) knots 0 0 0 1 2 2 2
  line L215 (35.5919, 13.323) -> (35.2008, 13.323)
  line L216 (35.2008, 13.323) -> (35.2008, 13.3395)
  spline S163 degree 2 poles (35.2008, 13.3395) (35.3326, 13.4568) (35.5981, 13.8005) (35.6969, 14.0064) knots 0 0 0 1 2 2 2
  spline S164 degree 2 poles (35.6969, 14.0064) (35.8039, 14.2266) (35.9274, 14.7165) (35.9274, 15.0005) knots 0 0 0 1 2 2 2
  spline S165 degree 2 poles (35.9274, 15.0005) (35.9274, 15.2825) (35.8019, 15.7827) (35.6969, 15.9947) knots 0 0 0 1 2 2 2
  spline S166 degree 2 poles (35.6969, 15.9947) (35.594, 16.2067) (35.3305, 16.5443) (35.2008, 16.6616) knots 0 0 0 1 2 2 2
  line L217 (35.2008, 16.6616) -> (35.2008, 16.6781)
  line L218 (35.2008, 16.6781) -> (35.5919, 16.6781)
  spline S167 degree 2 poles (35.5919, 16.6781) (35.8883, 16.3261) (36.228, 15.5316) (36.228, 15.0005) knots 0 0 0 1 2 2 2
  spline S168 degree 2 poles (3.5805, 6.9308) (3.5805, 6.2474) (3.1833, 5.6073) (2.7695, 5.6073) knots 0 0 0 1 2 2 2
  spline S169 degree 2 poles (2.7695, 5.6073) (2.3496, 5.6073) (1.9565, 6.2598) (1.9565, 6.9287) knots 0 0 0 1 2 2 2
  spline S170 degree 2 poles (1.9565, 6.9287) (1.9565, 7.6162) (2.3537, 8.2523) (2.7695, 8.2523) knots 0 0 0 1 2 2 2
  spline S171 degree 2 poles (2.7695, 8.2523) (3.1874, 8.2523) (3.5805, 7.5936) (3.5805, 6.9308) knots 0 0 0 1 2 2 2
  spline S172 degree 2 poles (3.1441, 6.1569) (3.1935, 6.2824) (3.2347, 6.6694) (3.2347, 6.9308) knots 0 0 0 1 2 2 2
  spline S173 degree 2 poles (3.2347, 6.9308) (3.2347, 7.1922) (3.1935, 7.5771) (3.1421, 7.7068) knots 0 0 0 1 2 2 2
  spline S174 degree 2 poles (3.1421, 7.7068) (3.0906, 7.8365) (2.9116, 7.9703) (2.7695, 7.9703) knots 0 0 0 1 2 2 2
  spline S175 degree 2 poles (2.7695, 7.9703) (2.6275, 7.9703) (2.4443, 7.8365) (2.3908, 7.7027) knots 0 0 0 1 2 2 2
  spline S176 degree 2 poles (2.3908, 7.7027) (2.3393, 7.573) (2.3023, 7.1778) (2.3023, 6.9287) knots 0 0 0 1 2 2 2
  spline S177 degree 2 poles (2.3023, 6.9287) (2.3023, 6.6612) (2.3352, 6.303) (2.3887, 6.163) knots 0 0 0 1 2 2 2
  spline S178 degree 2 poles (2.3887, 6.163) (2.4381, 6.0313) (2.6213, 5.8893) (2.7695, 5.8893) knots 0 0 0 1 2 2 2
  spline S179 degree 2 poles (2.7695, 5.8893) (2.9095, 5.8893) (3.0927, 6.0231) (3.1441, 6.1569) knots 0 0 0 1 2 2 2
  spline S180 degree 2 poles (4.6735, 5.6032) (4.4841, 5.6032) (4.1733, 5.7164) (4.0642, 5.8214) knots 0 0 0 1 2 2 2
  spline S181 degree 2 poles (4.0642, 5.8214) (3.9572, 5.9243) (3.846, 6.2042) (3.846, 6.3627) knots 0 0 0 1 2 2 2
  spline S182 degree 2 poles (3.846, 6.3627) (3.846, 6.5685) (4.0663, 6.9143) (4.2762, 7.0173) knots 0 0 0 1 2 2 2
  line L219 (4.2762, 7.0173) -> (4.2762, 7.0275)
  spline S183 degree 2 poles (4.2762, 7.0275) (4.0889, 7.1366) (3.9078, 7.396) (3.9078, 7.5895) knots 0 0 0 1 2 2 2
  spline S184 degree 2 poles (3.9078, 7.5895) (3.9078, 7.8756) (4.34, 8.2584) (4.6735, 8.2584) knots 0 0 0 1 2 2 2
  spline S185 degree 2 poles (4.6735, 8.2584) (5.0193, 8.2584) (5.4371, 7.8962) (5.4371, 7.6121) knots 0 0 0 1 2 2 2
  spline S186 degree 2 poles (5.4371, 7.6121) (5.4371, 7.4413) (5.2375, 7.1078) (5.0502, 7.0131) knots 0 0 0 1 2 2 2
  line L220 (5.0502, 7.0131) -> (5.0502, 7.0028)
  spline S187 degree 2 poles (5.0502, 7.0028) (5.2725, 6.8999) (5.501, 6.6035) (5.501, 6.3689) knots 0 0 0 1 2 2 2
  spline S188 degree 2 poles (5.501, 6.3689) (5.501, 6.0437) (5.0275, 5.6032) (4.6735, 5.6032) knots 0 0 0 1 2 2 2
  spline S189 degree 2 poles (5.151, 6.3359) (5.151, 6.4924) (5.0275, 6.6776) (4.8526, 6.7723) knots 0 0 0 1 2 2 2
  spline S190 degree 2 poles (4.8526, 6.7723) (4.7949, 6.8052) (4.6015, 6.8814) (4.48, 6.9308) knots 0 0 0 1 2 2 2
  spline S191 degree 2 poles (4.48, 6.9308) (4.34, 6.8382) (4.1898, 6.5624) (4.1898, 6.3874) knots 0 0 0 1 2 2 2
  spline S192 degree 2 poles (4.1898, 6.3874) (4.1898, 6.1569) (4.4677, 5.8563) (4.6776, 5.8563) knots 0 0 0 1 2 2 2
  spline S193 degree 2 poles (4.6776, 5.8563) (4.8917, 5.8563) (5.151, 6.1136) (5.151, 6.3359) knots 0 0 0 1 2 2 2
  spline S194 degree 2 poles (5.1037, 7.608) (5.1037, 7.7788) (4.8752, 8.0073) (4.6714, 8.0073) knots 0 0 0 1 2 2 2
  spline S195 degree 2 poles (4.6714, 8.0073) (4.4862, 8.0073) (4.2495, 7.8035) (4.2495, 7.6286) knots 0 0 0 1 2 2 2
  spline S196 degree 2 poles (4.2495, 7.6286) (4.2495, 7.503) (4.3709, 7.3281) (4.4924, 7.2581) knots 0 0 0 1 2 2 2
  spline S197 degree 2 poles (4.4924, 7.2581) (4.5438, 7.2293) (4.762, 7.1284) (4.8505, 7.0996) knots 0 0 0 1 2 2 2
  spline S198 degree 2 poles (4.8505, 7.0996) (4.9987, 7.2128) (5.1037, 7.4536) (5.1037, 7.608) knots 0 0 0 1 2 2 2
  line L221 (6.8677, 8.314) -> (5.8735, 5.1092)
  line L222 (5.8735, 5.1092) -> (5.5853, 5.1092)
  line L223 (5.5853, 5.1092) -> (6.5754, 8.314)
  line L224 (6.5754, 8.314) -> (6.8677, 8.314)
  line L225 (8.5864, 5.6608) -> (7.3473, 5.6608)
  line L226 (7.3473, 5.6608) -> (7.3473, 5.9202)
  line L227 (7.3473, 5.9202) -> (7.8084, 5.9202)
  line L228 (7.8084, 5.9202) -> (7.8084, 7.6224)
  line L229 (7.8084, 7.6224) -> (7.3473, 7.6224)
  line L230 (7.3473, 7.6224) -> (7.3473, 7.855)
  spline S199 degree 2 poles (7.3473, 7.855) (7.6087, 7.855) (7.8557, 8.0032) (7.8722, 8.209) knots 0 0 0 1 2 2 2
  line L231 (7.8722, 8.209) -> (8.1356, 8.209)
  line L232 (8.1356, 8.209) -> (8.1356, 5.9202)
  line L233 (8.1356, 5.9202) -> (8.5864, 5.9202)
  line L234 (8.5864, 5.9202) -> (8.5864, 5.6608)
  spline S200 degree 2 poles (9.7391, 7.96) (9.6465, 7.96) (9.4633, 7.9147) (9.3748, 7.8797) knots 0 0 0 1 2 2 2
  spline S201 degree 2 poles (9.3748, 7.8797) (9.2924, 7.8447) (9.171, 7.7706) (9.1236, 7.7377) knots 0 0 0 1 2 2 2
  line L235 (9.1236, 7.7377) -> (9.1031, 7.7377)
  line L236 (9.1031, 7.7377) -> (9.1031, 8.0979)
  spline S202 degree 2 poles (9.1031, 8.0979) (9.2142, 8.1576) (9.595, 8.2543) (9.7658, 8.2543) knots 0 0 0 1 2 2 2
  spline S203 degree 2 poles (9.7658, 8.2543) (9.9388, 8.2543) (10.196, 8.1843) (10.301, 8.1102) knots 0 0 0 1 2 2 2
  spline S204 degree 2 poles (10.301, 8.1102) (10.4122, 8.03) (10.5274, 7.7974) (10.5274, 7.6409) knots 0 0 0 1 2 2 2
  spline S205 degree 2 poles (10.5274, 7.6409) (10.5274, 7.431) (10.2516, 7.114) (10.0581, 7.0728) knots 0 0 0 1 2 2 2
  line L237 (10.0581, 7.0728) -> (10.0581, 7.0481)
  spline S206 degree 2 poles (10.0581, 7.0481) (10.1384, 7.0317) (10.3216, 6.9576) (10.3998, 6.8835) knots 0 0 0 1 2 2 2
  spline S207 degree 2 poles (10.3998, 6.8835) (10.478, 6.8114) (10.5768, 6.5809) (10.5768, 6.4142) knots 0 0 0 1 2 2 2
  spline S208 degree 2 poles (10.5768, 6.4142) (10.5768, 6.2433) (10.4595, 5.9531) (10.3525, 5.8419) knots 0 0 0 1 2 2 2
  spline S209 degree 2 poles (10.3525, 5.8419) (10.2413, 5.7267) (9.9264, 5.6073) (9.7267, 5.6073) knots 0 0 0 1 2 2 2
  spline S210 degree 2 poles (9.7267, 5.6073) (9.5353, 5.6073) (9.1607, 5.6999) (9.0331, 5.7637) knots 0 0 0 1 2 2 2
  line L238 (9.0331, 5.7637) -> (9.0331, 6.1239)
  line L239 (9.0331, 6.1239) -> (9.0578, 6.1239)
  spline S211 degree 2 poles (9.0578, 6.1239) (9.1648, 6.0457) (9.5271, 5.9016) (9.7062, 5.9016) knots 0 0 0 1 2 2 2
  spline S212 degree 2 poles (9.7062, 5.9016) (9.8111, 5.9016) (10.0211, 5.9675) (10.0911, 6.0437) knots 0 0 0 1 2 2 2
  spline S213 degree 2 poles (10.0911, 6.0437) (10.159, 6.1198) (10.231, 6.301) (10.231, 6.4389) knots 0 0 0 1 2 2 2
  spline S214 degree 2 poles (10.231, 6.4389) (10.231, 6.5768) (10.1508, 6.7558) (10.0787, 6.8073) knots 0 0 0 1 2 2 2
  spline S215 degree 2 poles (10.0787, 6.8073) (10.0067, 6.8588) (9.8111, 6.8979) (9.6959, 6.8979) knots 0 0 0 1 2 2 2
  line L240 (9.6959, 6.8979) -> (9.5518, 6.8979)
  line L241 (9.5518, 6.8979) -> (9.5518, 7.1799)
  line L242 (9.5518, 7.1799) -> (9.665, 7.1799)
  spline S216 degree 2 poles (9.665, 7.1799) (9.8935, 7.1799) (10.1816, 7.3981) (10.1816, 7.6059) knots 0 0 0 1 2 2 2
  spline S217 degree 2 poles (10.1816, 7.6059) (10.1816, 7.7027) (10.1075, 7.8406) (10.0478, 7.8818) knots 0 0 0 1 2 2 2
  spline S218 degree 2 poles (10.0478, 7.8818) (9.984, 7.925) (9.8276, 7.96) (9.7391, 7.96) knots 0 0 0 1 2 2 2
  line L243 (12.0156, 8.314) -> (11.0214, 5.1092)
  line L244 (11.0214, 5.1092) -> (10.7333, 5.1092)
  line L245 (10.7333, 5.1092) -> (11.7233, 8.314)
  line L246 (11.7233, 8.314) -> (12.0156, 8.314)
  line L247 (13.862, 5.6608) -> (12.2956, 5.6608)
  line L248 (12.2956, 5.6608) -> (12.2956, 6.021)
  spline S219 degree 2 poles (12.2956, 6.021) (12.4643, 6.1795) (12.7649, 6.4739) (12.9089, 6.6323) knots 0 0 0 1 2 2 2
  spline S220 degree 2 poles (12.9089, 6.6323) (13.1992, 6.9514) (13.4112, 7.3342) (13.4112, 7.538) knots 0 0 0 1 2 2 2
  spline S221 degree 2 poles (13.4112, 7.538) (13.4112, 7.6451) (13.3453, 7.8056) (13.2856, 7.8571) knots 0 0 0 1 2 2 2
  spline S222 degree 2 poles (13.2856, 7.8571) (13.2259, 7.9085) (13.0695, 7.96) (12.9748, 7.96) knots 0 0 0 1 2 2 2
  spline S223 degree 2 poles (12.9748, 7.96) (12.8842, 7.96) (12.699, 7.9147) (12.6146, 7.8797) knots 0 0 0 1 2 2 2
  spline S224 degree 2 poles (12.6146, 7.8797) (12.5426, 7.8509) (12.4088, 7.7686) (12.3676, 7.7397) knots 0 0 0 1 2 2 2
  line L249 (12.3676, 7.7397) -> (12.3491, 7.7397)
  line L250 (12.3491, 7.7397) -> (12.3491, 8.102)
  spline S225 degree 2 poles (12.3491, 8.102) (12.454, 8.1535) (12.8307, 8.2543) (12.9995, 8.2543) knots 0 0 0 1 2 2 2
  spline S226 degree 2 poles (12.9995, 8.2543) (13.3556, 8.2543) (13.757, 7.8776) (13.757, 7.5565) knots 0 0 0 1 2 2 2
  spline S227 degree 2 poles (13.757, 7.5565) (13.757, 7.4063) (13.687, 7.1552) (13.6252, 7.0481) knots 0 0 0 1 2 2 2
  spline S228 degree 2 poles (13.6252, 7.0481) (13.5635, 6.937) (13.3844, 6.7188) (13.2856, 6.6138) knots 0 0 0 1 2 2 2
  spline S229 degree 2 poles (13.2856, 6.6138) (13.1251, 6.4389) (12.7319, 6.0642) (12.6146, 5.9551) knots 0 0 0 1 2 2 2
  line L251 (12.6146, 5.9551) -> (13.862, 5.9551)
  line L252 (13.862, 5.9551) -> (13.862, 5.6608)
  spline S230 degree 2 poles (15.7412, 6.4677) (15.7412, 6.2845) (15.6239, 5.9716) (15.5169, 5.8563) knots 0 0 0 1 2 2 2
  spline S231 degree 2 poles (15.5169, 5.8563) (15.4098, 5.7411) (15.0908, 5.6073) (14.8932, 5.6073) knots 0 0 0 1 2 2 2
  spline S232 degree 2 poles (14.8932, 5.6073) (14.7121, 5.6073) (14.358, 5.6876) (14.2283, 5.7514) knots 0 0 0 1 2 2 2
  line L253 (14.2283, 5.7514) -> (14.2283, 6.1116)
  line L254 (14.2283, 6.1116) -> (14.253, 6.1116)
  spline S233 degree 2 poles (14.253, 6.1116) (14.2922, 6.0828) (14.4383, 6.0087) (14.5268, 5.9757) knots 0 0 0 1 2 2 2
  spline S234 degree 2 poles (14.5268, 5.9757) (14.6277, 5.9407) (14.7944, 5.9016) (14.8994, 5.9016) knots 0 0 0 1 2 2 2
  spline S235 degree 2 poles (14.8994, 5.9016) (15.0023, 5.9016) (15.1958, 5.9757) (15.2658, 6.056) knots 0 0 0 1 2 2 2
  spline S236 degree 2 poles (15.2658, 6.056) (15.3296, 6.1322) (15.3954, 6.3339) (15.3954, 6.4697) knots 0 0 0 1 2 2 2
  spline S237 degree 2 poles (15.3954, 6.4697) (15.3954, 6.6056) (15.3213, 6.7785) (15.2513, 6.8361) knots 0 0 0 1 2 2 2
  spline S238 degree 2 poles (15.2513, 6.8361) (15.1793, 6.8999) (14.9652, 6.9534) (14.8356, 6.9534) knots 0 0 0 1 2 2 2
  spline S239 degree 2 poles (14.8356, 6.9534) (14.6956, 6.9534) (14.4177, 6.9102) (14.3333, 6.8917) knots 0 0 0 1 2 2 2
  line L255 (14.3333, 6.8917) -> (14.3333, 8.2008)
  line L256 (14.3333, 8.2008) -> (15.7268, 8.2008)
  line L257 (15.7268, 8.2008) -> (15.7268, 7.9023)
  line L258 (15.7268, 7.9023) -> (14.6606, 7.9023)
  line L259 (14.6606, 7.9023) -> (14.6606, 7.2251)
  spline S240 degree 2 poles (14.6606, 7.2251) (14.7223, 7.2334) (14.8417, 7.2396) (14.8911, 7.2396) knots 0 0 0 1 2 2 2
  spline S241 degree 2 poles (14.8911, 7.2396) (15.0867, 7.2396) (15.3563, 7.1757) (15.4798, 7.0811) knots 0 0 0 1 2 2 2
  spline S242 degree 2 poles (15.4798, 7.0811) (15.6054, 6.9864) (15.7412, 6.6982) (15.7412, 6.4677) knots 0 0 0 1 2 2 2
  point P0 (44, -10)
  dimension "d0" = 115
  dimension "d1" = 115
  constraints: 2 other
extrude "Extrusion3" cut sketch "Sketch6" against normal blind 2
equation "\"d153\" = d124"
equation "\"d124\" = 34.641016"
body "Solid1"
